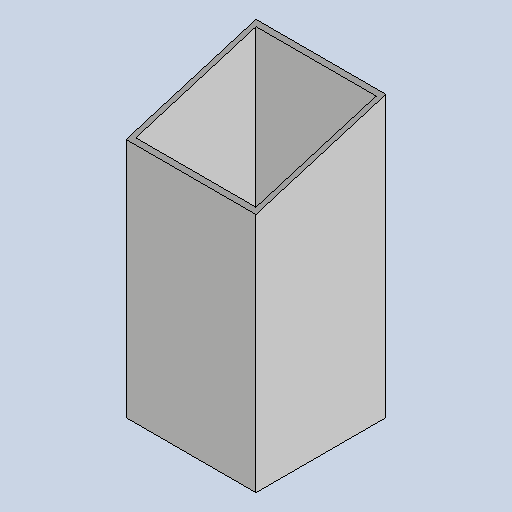
# Autodesk Inventor part: TZS 1284 leg tube
Saved by Autodesk Inventor 2025 (Build 290162010, 162A)
## iProperties
Created: 2025-07-17
Part Number: TZS 1284 leg tube
Material: Generic
Document SubType Name: Modeling
Designer: admin
Density: 1 g/cm^3
Appearance: Default
Author: admin
Autodesk Inventor part; units mm, degrees
ref_plane "YZ Plane" through (0, 0, 0) normal (1, 0, 0) x (0, 1, 0)
ref_plane "XZ Plane" through (0, 0, 0) normal (0, 1, 0) x (-1, 0, 0)
ref_plane "XY Plane" through (0, 0, 0) normal (0, 0, 1) x (1, 0, 0)
sketch "Sketch1" plane through (0, 0, 0) normal (0, 0, 1) x (1, 0, 0)
  line L0 (40, -40) -> (-40, -40)
  line L1 (-40, -40) -> (-40, 40)
  line L2 (-40, 40) -> (40, 40)
  line L3 (40, 40) -> (40, -40)
  line L4 (40, -40) -> (-40, 40) construction
  line L5 (-40, -40) -> (40, 40) construction
  line L6 (-37, -37) -> (37, -37)
  line L7 (37, -37) -> (37, 37)
  line L8 (37, 37) -> (-37, 37)
  line L9 (-37, 37) -> (-37, -37)
  point P0 (0, 0)
  dimension "d0" = 80
  dimension "d1" = 80
  dimension "d2" = 3
  constraints: 20 end point, 4 parallel, 2 midpoint, 2 perpendicular, 1 horizontal, 3 other
  measures "d0" distance of L1.end L2.end
  measures "d1" distance of L0.end L1.end
  measures "d2" distance between parallel lines of L0 L6
extrude "Extrusion1" add sketch "Sketch1" along normal blind 172.4121
sketch "Sketch2" plane through (0, 0, 0) normal (1, 0, 0) x (0, 1, 0)
  line L0 (40, 0) -> (-40, 0) projected
  line L1 (-40, 0) -> (-40, 172.4121) projected
  line L2 (40, 172.4121) -> (-40, 172.4121) projected
  line L3 (40, 0) -> (40, 172.4121) projected
  line L4 (40, 172.4121) -> (-40, 148.3319)
  point P0 (0, 0)
  dimension "d5" = 16.752
  constraints: 2 end point, 1 point on line
  measures "d5" angle of L4 L2
extrude "Extrusion2" cut sketch "Sketch2" along normal through all both and the other way through all contours L4 L1 L2
equation "\"d3\" = Lenth"
equation "\"d5\" = Leg_cut_angle"
equation "\"Lenth\" = Leg_hight"
equation "\"Leg_cut_angle\" = 16.751975deg"
equation "\"Leg_hight\" = 172.412142"
body "Solid1"
